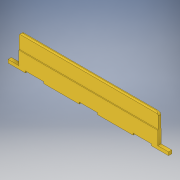
# Autodesk Inventor part: QTE-T-1G1-01_imp
Saved by Autodesk Inventor 2019 (Build 230136000, 136)
## iProperties
Created: 2024-08-20
Part Number: QTE-T-1G1-01_imp
Material: Generic
Catalog Web Link: www.cadenas.de
Description: QTE Series Integral Metal Plane for Power or Ground-QTE Series - (0,80 mm) .0315" Q Strip® High Speed Ground Plane Header
Vendor: SAMTEC
Document SubType Name: Modeling
Designer: psAdmin
Manufacturer: SAMTEC
Mass: 0.0208165 g
Surface Area: 1.36415 cm^2
Volume: 0.0208165 cm^3
Density: 1 g/cm^3
Appearance: PSOLRGB-212-179-45
Category: PARTsolutions
Company: SAMTEC
Title: QTE-T-1G1-01_imp
Author: Cadenas PARTsolutions
Comments: QTE Series - (0,80 mm) .0315" Q Strip® High Speed Ground Plane Header
PSOL_IDENT_0: {$CADENAS_DATA/23d-libs/samtec/modelling/qte/parts/qte_integral_metal_plane_for_power_or_ground.prj}
PSOL_IDENT_1: ,219 {VTYP=3D},{NB=QTE-T-1G1-01_imp},{LINA=QTE-T-1G1-01_imp},{NN=QTE Series Integral Metal Plane for
PSOL_IDENT_2: Power or Ground},{DATE=13.08.2024 10:44:10},{GEOMDATE=16.03.2016 08:37:00},{VERSION=},{LINEID=10},{
PSOL_IDENT_3: WBVAR=LS},{WBNUMERIC=}  {NB=QTE-T-1G1-01_imp},{LINA=QTE-T-1G1-01_imp},{KT=DUMMY},{PN=T-1G1-01},{SERI
PSOL_IDENT_4: ES=QTE},{LS=01},{LSALG= '01', '-01', '02', '-02', '03', '-03', '04', '-04', '05', '-05'  ,'06','-06'
PSOL_IDENT_5: , '07', '-07' ,'08','-08','09','-09','10','-10' },{A=0.1680},{H=0.1970},{CH=0.1600}
NB: QTE-T-1G1-01_imp
NN: QTE Series Integral Metal Plane for Power or Ground
NT: QTE Series - (0,80 mm) .0315" Q Strip® High Speed Ground Plane Header
NBSYN: QTE-$PN._imp
LINA: QTE-T-1G1-01_imp
CATALOG: Samtec
SERIES: QTE
LS: -01
SUPPLIER: SAMTEC
ARTICLENO: QTE-T-1G1-01_imp
BOMINFO: QTE-T-1G1-01_imp
CREATOR: CADENAS GmbH
Autodesk Inventor part; units mm, degrees
sketch "Sketch_1" plane through (0, 0, 0) normal (0, 0, 1) x (1, 0, 0)
  line L0 (-9.4615, 0.1778) -> (-9.4615, -0.2032)
  line L1 (-9.4615, -0.2032) -> (-7.429, -0.2032)
  line L2 (-7.429, -0.2032) -> (-7.429, 0)
  line L3 (-7.429, 0) -> (-5.271, 0)
  line L4 (-5.271, 0) -> (-5.271, -0.203)
  line L5 (-5.271, -0.203) -> (-1.08, -0.203)
  line L6 (-1.08, -0.203) -> (-1.08, 0)
  line L7 (-1.08, 0) -> (1.08, 0)
  line L8 (1.08, 0) -> (1.08, -0.2032)
  line L9 (1.08, -0.2032) -> (5.27, -0.2032)
  line L10 (5.27, -0.2032) -> (5.27, 0)
  line L11 (5.27, 0) -> (7.429, 0)
  line L12 (7.429, 0) -> (7.429, -0.2032)
  line L13 (7.429, -0.2032) -> (9.4615, -0.2032)
  line L14 (9.4615, -0.2032) -> (9.4615, 0.1778)
  line L15 (9.4615, 0.1778) -> (8.1915, 0.1778)
  line L16 (8.1915, 0.1778) -> (8.1915, 3.175)
  arc A0 (8.1915, 3.175) -> (7.8105, 3.556) centre (7.8105, 3.175) ccw
  line L17 (7.8105, 3.556) -> (-7.8105, 3.556)
  arc A1 (-7.8105, 3.556) -> (-8.1915, 3.175) centre (-7.8105, 3.175) ccw
  line L18 (-8.1915, 3.175) -> (-8.1915, 0.1778)
  line L19 (-8.1915, 0.1778) -> (-9.4615, 0.1778)
  constraints: 40 end point, 4 point on circle, 2 centre point
extrude "Extrusion1" add sketch "Sketch_1" along normal mid plane 0.8
sketch "Sketch_2" plane through (0, 0, 0) normal (1, 0, 0) x (0, 1, 0)
  line L0 (-8.5344, 8.5344) -> (-8.5344, -8.5344)
  line L1 (-8.5344, -8.5344) -> (8.5344, -8.5344)
  line L2 (8.5344, -8.5344) -> (8.5344, 8.5344)
  line L3 (8.5344, 8.5344) -> (-8.5344, 8.5344)
  line L4 (1.7526, 0.1905) -> (-0.2032, 0.1905)
  line L5 (-0.2032, 0.1905) -> (-0.2032, -0.1905)
  line L6 (-0.2032, -0.1905) -> (1.7526, -0.1905)
  line L7 (1.7526, -0.1905) -> (1.8186, -0.1524)
  line L8 (1.8186, -0.1524) -> (3.38, -0.1524)
  line L9 (3.38, -0.1524) -> (3.556, -0.0508)
  line L10 (3.556, -0.0508) -> (3.556, 0.0508)
  line L11 (3.556, 0.0508) -> (3.38, 0.1524)
  line L12 (3.38, 0.1524) -> (1.8186, 0.1524)
  line L13 (1.8186, 0.1524) -> (1.7526, 0.1905)
  constraints: 28 end point
extrude "Extrusion2" cut sketch "Sketch_2" along normal mid plane 20
ref_plane "integral_metal_plane_XY" through (0, -0.2032, 0) normal (0, 1, 0) x (1, 0, 0)
ref_plane "integral_metal_plane_YZ" through (0, -0.2032, 0) normal (1, 0, 0) x (0, 0, -1)
ref_plane "integral_metal_plane_ZX" through (0, -0.2032, 0) normal (0, 0, -1) x (0, 1, 0)
body "Solid1"
